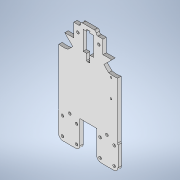
# Autodesk Inventor part: Основа робота
Saved by Autodesk Inventor 2020 (Build 240168000, 168)
## iProperties
Created: 2021-02-28
Part Number: Основа робота
Material: Типовые
Document SubType Name: Обычные детали
Designer: Антон
Density: 1 g/cm^3
Appearance: По умолчанию
Mass: 52.0111 g
Surface Area: 352.197 cm^2
Volume: 52.0111 cm^3
Sheet Metal Rule: По умолчанию
Author: Антон
Autodesk Inventor part; units mm, degrees
note: some values were not read from the file. Chosen so that the rebuilt part matches the saved one: direction of "Рельеф1".
ref_plane "YZ Plane" through (0, 0, 0) normal (1, 0, 0) x (0, 1, 0)
ref_plane "XZ Plane" through (0, 0, 0) normal (0, 1, 0) x (-1, 0, 0)
ref_plane "XY Plane" through (0, 0, 0) normal (0, 0, 1) x (1, 0, 0)
sketch "Эскиз1" plane through (0, 0, 0) normal (0, 0, 1) x (1, 0, 0)
  line L0 (0, 0) -> (35, 0)
  line L1 (35, 0) -> (35, 128.55)
  line L2 (35, 128.55) -> (0, 128.55)
  line L3 (0, 128.55) -> (0, 0)
  line L4 (0, 0) -> (-0.3, 0)
  line L5 (-0.3, 0) -> (-0.3, 30.3)
  line L6 (-0.3, 30.3) -> (0, 30.3)
  line L7 (0, 30.3) -> (0, 0)
  line L8 (-0.3, 0) -> (4.25, 0)
  line L9 (4.25, 0) -> (4.25, 4.55)
  line L10 (4.25, 4.55) -> (4.25, 25.75) construction
  circle A0 centre (4.25, 25.75) radius 1.6
  circle A1 centre (4.25, 4.55) radius 1.6
  line L11 (35, 0) -> (25, 0)
  line L12 (25, 0) -> (25, 33)
  line L13 (25, 33) -> (35, 33)
  line L14 (35, 33) -> (35, 0)
  line L15 (25, 4.55) -> (21, 4.55)
  line L16 (25, 25.75) -> (21, 25.75)
  circle A2 centre (21, 25.75) radius 1.6
  circle A3 centre (21, 4.55) radius 1.6
  line L17 (35, 128.55) -> (35, 128.55)
  line L18 (35, 128.55) -> (18, 128.55)
  line L19 (21, 25.75) -> (21, 4.55) construction
  circle A4 centre (22.55, 120.55) radius 1.6
  line L20 (17.6, 128.55) -> (17.6, 112.55)
  line L21 (17.6, 112.55) -> (0, 112.55)
  line L22 (0, 112.55) -> (0, 129.6)
  line L23 (35, 128.55) -> (25.75, 128.55)
  line L24 (25.75, 128.55) -> (25.75, 133)
  line L25 (25.75, 133) -> (35, 133)
  line L26 (35, 133) -> (35, 128.55)
  line L27 (17.6, 120.55) -> (5.05, 120.55) construction
  line L28 (5.05, 120.55) -> (-3.6474, 111.8526) construction
  line L29 (-3.6474, 111.8526) -> (10.8483, 97.3569)
  circle A5 centre (5.05, 120.55) radius 23.9069
  line L30 (0, 112.55) -> (13, 112.55)
  line L31 (13, 112.55) -> (13, 98.0037)
  line L32 (13, 98.0037) -> (0, 98.0037)
  line L33 (0, 98.0037) -> (0, 112.55)
  line L34 (-3.6474, 111.8526) -> (2.0094, 117.5094)
  line L35 (2.0094, 117.5094) -> (16.5051, 103.0138)
  line L36 (16.5051, 103.0138) -> (10.8483, 97.3569)
  line L37 (10.8483, 97.3569) -> (-3.6474, 111.8526)
  point P0 (0, 30.3)
  point P1 (25, 0)
  point P2 (0, 182.1)
  point P3 (21, 15.15)
  point P4 (4.25, 15.15)
  point P5 (11.6, 112.55)
  point P6 (0, 97.1826)
  point P7 (25.75, 132.5104)
  point P8 (27.5786, 128.55)
  point P9 (25.9614, 133)
  point P10 (27.5786, 128.55)
  point P11 (17.336, 116.55)
  point P12 (17.6, 116.9708)
  point P13 (17.6, 132.1292)
  point P14 (14.4448, 116.55)
  point P15 (0, 108.2052)
  point P16 (10.2015, 98.0037)
  point P17 (6.9689, 112.55)
  point P18 (13, 106.5189)
  point P19 (13, 99.5086)
  dimension "d0" = 35
  dimension "d1" = 128.55
  dimension "d191" = 0.3
  dimension "d192" = 30.3
  dimension "d207" = 4.55
  dimension "d208" = 4.55
  dimension "d209" = 21.2
  dimension "d210" = 10
  dimension "d211" = 33
  dimension "d215" = 4
  dimension "d290" = 3.2
  dimension "d387" = 21.2
  dimension "d418" = 4.55
  dimension "d421" = 3.2
  dimension "d427" = 17.6
  dimension "d428" = 16
  dimension "d433" = 4.95
  dimension "d448" = 9.25
  dimension "d450" = 4.45
  dimension "d493" = 12.55
  dimension "d494" = 12.3
  dimension "d495" = 20.5
  dimension "d496" = 13
  dimension "d499" = 135
  dimension "d500" = 8
  constraints: 76 end point, 14 parallel, 10 perpendicular, 8 horizontal, 7 point on line, 6 centre point, 5 coincident, 3 equal radius, 3 midpoint, 2 collinear, 2 horizontal alignment, 2 point on circle, 1 vertical
  measures "d0" distance of L2.end L1.end
  measures "d1" distance of L1.end L0.end
  measures "d191" distance of L5.end L6.end
  measures "d192" distance of L4.end L5.end
  measures "d207" distance of L4.end L8.end
  measures "d208" distance of L8.end L9.end
  measures "d209" distance of L9.end L10.end
  measures "d210" distance of L12.end L13.end
  measures "d211" distance of L11.end L12.end
  measures "d215" distance of L16.start L16.end
  measures "d290" diameter of A2
  measures "d387" distance of L19.end L19.start
  measures "d418" distance from line of L0 L15.end
  measures "d421" diameter of A4
  measures "d427" distance of L20.end L21.end
  measures "d428" distance of L20.start L20.end
  measures "d433" distance of A4.centre L27.start
  measures "d448" distance of L24.end L25.end
  measures "d450" distance of L23.end L24.end
  measures "d493" distance of L27.start L27.end
  measures "d494" distance of L27.end L28.end
  measures "d495" distance of L28.end L29.end
  measures "d496" distance of L31.end L32.end
  measures "d499" angle of L27 L28
  measures "d500" distance between parallel lines of L37 L35
extrude "Выдавливание1" add sketch "Эскиз1" along normal blind 4 contours L3 A5 L2 L1 L13 L12 L0 | L4 L5 L6 L3 | A5 L2 L24 | L24 L25 L26 L2 A5 | L36 L32 A5 | L2 A5 L31 L36 L35 L21 L20 | L32 L36 L31 | L21 L31 L35
mirror "Зеркальное отражение1" about plane through (35, 33, 0) normal (1, 0, 0)
sketch "Эскиз32" plane through (0, 0, 4) normal (0, 0, 1) x (1, 0, 0)
  line L0 (25, 33) -> (45, 33) projected
  line L1 (25, 0) -> (25, 33) construction
  line L2 (45, 0) -> (45, 33) construction
  line L3 (25, 0) -> (45, 0) construction
  line L4 (35, 0) -> (35, 32.3) construction
  line L5 (12.975, 32.3) -> (57.025, 32.3) construction
  dimension "d501" = 32.3
  dimension "d502" = 44.05
  constraints: 6 end point, 2 midpoint, 1 horizontal, 1 perpendicular, 1 vertical
  measures "d501" distance of L4.start L4.end
  measures "d502" distance of L5.start L5.end
hole "Отверстие14" at (12.975, 32.3, 4) at (57.025, 32.3, 4) direction (0, 0, -1) diameter 3.2 end through all
sketch "Эскиз35" plane through (0, 0, 4) normal (0, 0, 1) x (1, 0, 0)
  line L0 (25.75, 133) -> (44.25, 133) construction
  line L1 (35, 133) -> (35, 83) construction
  line L2 (35, 83) -> (62, 83) construction
  line L3 (62, 72) -> (62, 94) construction
  point P0 (0, 0)
  dimension "d503" = 50
  dimension "d504" = 27
  dimension "d505" = 22
  constraints: 6 end point, 2 midpoint, 2 vertical, 1 horizontal
  measures "d503" distance of L1.start L1.end
  measures "d504" distance of L2.end L1.end
  measures "d505" distance of L3.start L3.end
hole "Отверстие16" at (62, 72, 4) at (62, 94, 4) direction (0, 0, -1) diameter 2.2 end through all
sketch "Эскиз33" plane through (0, 0, 4) normal (0, 0, 1) x (1, 0, 0)
  line L0 (25.75, 133) -> (35, 133) construction
  line L1 (35, 133) -> (35, 129) construction
  line L2 (41.25, 127) -> (28.75, 127)
  line L3 (28.75, 127) -> (28.75, 104.2)
  line L4 (28.75, 104.2) -> (41.25, 104.2)
  line L5 (41.25, 104.2) -> (41.25, 127)
  line L6 (33, 129) -> (37, 129)
  line L7 (37, 129) -> (37, 127)
  line L8 (37, 127) -> (33, 127)
  line L9 (33, 127) -> (33, 129)
  line L10 (33, 104.2) -> (37, 104.2)
  line L11 (37, 104.2) -> (37, 96)
  line L12 (37, 96) -> (33, 96)
  line L13 (33, 96) -> (33, 104.2)
  point P0 (0, 0)
  point P1 (44.25, 133)
  point P2 (35, 127)
  point P3 (35, 104.2)
  point P4 (37, 127)
  point P5 (33, 127)
  point P6 (26.4635, 133)
  dimension "d465" = 12.5
  dimension "d466" = 22.8
  dimension "d467" = 2
  dimension "d468" = 4
  dimension "d469" = 4
  dimension "d470" = 4
  dimension "d471" = 8.2
  constraints: 27 end point, 6 parallel, 5 midpoint, 3 horizontal, 3 perpendicular, 1 vertical
  measures "d465" distance between parallel lines of L5 L3
  measures "d466" distance of L4.end L2.start
  measures "d467" distance of L6.end L7.end
  measures "d468" distance of L6.start L6.end
  measures "d469" distance of L0.end L1.end
  measures "d470" distance of L11.end L12.end
  measures "d471" distance of L10.end L11.end
extrude "Выдавливание14" cut sketch "Эскиз33" against normal through all
fillet "Сопряжение14" radius 1 2 edges at (37, 96, 2) (33, 96, 2)
fillet "Сопряжение13" radius 2.225 4 edges at (25.75, 128.55, 2) (25.75, 133, 2) (44.25, 128.55, 2) (44.25, 133, 2)
fillet "Сопряжение2" radius 5.05 6 edges at (-0.3, 30.3, 2) (-0.3, 0, 2) (25, 0, 2) (45, 0, 2) (70.3, 0, 2) (70.3, 30.3, 2)
sketch "Эскиз19" plane through (0, 0, 0) normal (0, 0, -1) x (-1, 0, 0)
  line L0 (-25.75, 128.55) -> (-17.6, 128.55) projected
  line L1 (-25.35, 122.1666) -> (-22.55, 123.7832)
  line L2 (-22.55, 123.7832) -> (-19.75, 122.1666)
  line L3 (-19.75, 122.1666) -> (-19.75, 118.9334)
  line L4 (-19.75, 118.9334) -> (-22.55, 117.3168)
  line L5 (-22.55, 117.3168) -> (-25.35, 118.9334)
  line L6 (-25.35, 118.9334) -> (-25.35, 122.1666)
  line L7 (0, 97.1826) -> (0, 30.3) projected
  circle A0 centre (-22.55, 120.55) radius 1.6 projected
  point P0 (0, 128.55)
  point P1 (-70, 128.55)
  point P2 (-14, 129.6)
  point P3 (-64, 129.6)
  point P4 (0, 119.25)
  point P5 (0, 116.55)
  point P6 (0, 129.6)
  point P7 (-78, 129.6)
  point P8 (-17.6, 128.55)
  point P9 (-52.4, 128.55)
  point P10 (0, 107.125)
  point P11 (-35, 132.55)
  point P12 (-27.0423, 128.55)
  point P13 (0, 0)
  point P14 (0, 102.0037)
  dimension "d423" = 5.6
  constraints: 12 end point, 1 coincident, 1 vertical, 15 other
  measures "d423" distance between parallel lines of L3 L6
extrude "Выдавливание7" cut sketch "Эскиз19" against normal blind 2.6 contours L1 L2 L3 L4 L5 L6 | A0
sketch "Эскиз25" plane through (0, 0, 0) normal (0, 0, -1) x (-1, 0, 0)
  circle A0 centre (-21, 25.75) radius 1.6 projected
  circle A1 centre (-21, 4.55) radius 1.6 projected
  circle A2 centre (-4.25, 25.75) radius 1.6 projected
  circle A3 centre (-4.25, 4.55) radius 1.6 projected
  circle A4 centre (-49, 25.75) radius 1.6 projected
  circle A5 centre (-49, 4.55) radius 1.6 projected
  circle A6 centre (-65.75, 4.55) radius 1.6 projected
  circle A7 centre (-65.75, 25.75) radius 1.6 projected
  circle A8 centre (-47.45, 120.55) radius 1.6 projected
  circle A9 centre (-47.45, 120.55) radius 1.6 projected
  circle A10 centre (-57.025, 32.3) radius 1.6 projected
  circle A11 centre (-12.975, 32.3) radius 1.6 projected
  circle A12 centre (-57.025, 32.3) radius 1.6 projected
  circle A13 centre (-12.975, 32.3) radius 1.6 projected
  point P0 (0, 0)
  constraints: 12 coincident
pattern_sketch "Массив по эскизу1" of "Выдавливание7" from (22.55, 120.55, 0) copies at (21, 25.75, 0) at (21, 4.55, 0) at (4.25, 25.75, 0) at (4.25, 4.55, 0) at (49, 25.75, 0) at (49, 4.55, 0) at (65.75, 4.55, 0) at (65.75, 25.75, 0) at (47.45, 120.55, 0) at (57.025, 32.3, 0) at (12.975, 32.3, 0)
sketch "Эскиз31" plane through (0, 0, 0) normal (0, 0, -1) x (-1, 0, 0)
  line L0 (-70, 96.6431) -> (0, 96.6431) construction
  line L1 (0, 96.6431) -> (0, 33) construction
  line L2 (0, 33) -> (-70, 33) construction
  line L3 (-70, 33) -> (-70, 96.6431) construction
  line L4 (0, 97.1826) -> (0, 30.3) projected
  line L5 (-70, 97.1826) -> (-70, 30.3) projected
  line L6 (-25, 33) -> (-45, 33) projected
  arc A0 (-10.8483, 97.3569) -> (0, 97.1826) centre (-5.05, 120.55) ccw projected
  line L7 (-43.3655, 68.2237) -> (-41.8166, 72.9961)
  line L8 (-41.8166, 72.9961) -> (-40.6499, 72.9961)
  line L9 (-40.6499, 72.9961) -> (-42.8475, 66.8961)
  line L10 (-42.8475, 66.8961) -> (-43.8734, 66.8961)
  line L11 (-43.8734, 66.8961) -> (-46.061, 72.9961)
  line L12 (-46.061, 72.9961) -> (-44.8993, 72.9961)
  line L13 (-44.8993, 72.9961) -> (-43.3655, 68.2237)
  line L14 (-38.9803, 66.8961) -> (-39.9962, 66.8961)
  line L15 (-39.9962, 66.8961) -> (-39.9962, 71.4271)
  line L16 (-39.9962, 71.4271) -> (-38.9803, 71.4271)
  line L17 (-38.9803, 71.4271) -> (-38.9803, 66.8961)
  spline S0 degree 2 poles (-40.0615, 72.6038) (-40.0615, 72.8352) (-39.7648, 73.1469) (-39.2117, 73.1469) (-38.9099, 72.8352) (-38.9099, 72.6038) knots 0 0 0 1 2 3 4 4 4
  spline S1 degree 2 poles (-38.9099, 72.6038) (-38.9099, 72.3725) (-39.2117, 72.0657) (-39.7648, 72.0657) (-40.0615, 72.3725) (-40.0615, 72.6038) knots 0 0 0 1 2 3 4 4 4
  spline S2 degree 2 poles (-38.0601, 69.2043) (-38.0601, 69.8681) (-37.532, 70.9393) (-36.5765, 71.5126) (-35.958, 71.5126) knots 0 0 0 1 2 3 3 3
  spline S3 degree 2 poles (-35.958, 71.5126) (-35.0427, 71.5126) (-33.8962, 70.3308) (-33.8509, 69.3552) knots 0 0 0 1 2 2 2
  line L18 (-33.8509, 69.3552) -> (-33.8459, 69.1138)
  spline S4 degree 2 poles (-33.8459, 69.1138) (-33.8459, 68.445) (-34.3639, 67.3889) (-35.3244, 66.8106) (-35.9479, 66.8106) knots 0 0 0 1 2 3 3 3
  spline S5 degree 2 poles (-35.9479, 66.8106) (-36.9085, 66.8106) (-38.0601, 68.0879) (-38.0601, 69.154) knots 0 0 0 1 2 2 2
  line L19 (-38.0601, 69.154) -> (-38.0601, 69.2043)
  spline S6 degree 2 poles (-37.0442, 69.1188) (-37.0442, 68.4198) (-36.4659, 67.6253) (-35.435, 67.6253) (-34.8617, 68.4299) (-34.8617, 69.2043) knots 0 0 0 1 2 3 4 4 4
  spline S7 degree 2 poles (-34.8617, 69.2043) (-34.8617, 69.8933) (-35.4501, 70.6979) (-35.958, 70.6979) knots 0 0 0 1 2 2 2
  spline S8 degree 2 poles (-35.958, 70.6979) (-36.4559, 70.6979) (-37.0442, 69.9033) (-37.0442, 69.1188) knots 0 0 0 1 2 2 2
  line L20 (-31.9047, 66.8961) -> (-32.9206, 66.8961)
  line L21 (-32.9206, 66.8961) -> (-32.9206, 73.333)
  line L22 (-32.9206, 73.333) -> (-31.9047, 73.333)
  line L23 (-31.9047, 73.333) -> (-31.9047, 66.8961)
  spline S9 degree 2 poles (-28.8019, 66.8106) (-29.7675, 66.8106) (-30.9694, 68.0326) (-30.9694, 69.0434) knots 0 0 0 1 2 2 2
  line L24 (-30.9694, 69.0434) -> (-30.9694, 69.1691)
  spline S10 degree 2 poles (-30.9694, 69.1691) (-30.9694, 69.848) (-30.4464, 70.9192) (-29.5009, 71.5126) (-28.9176, 71.5126) knots 0 0 0 1 2 3 3 3
  spline S11 degree 2 poles (-28.9176, 71.5126) (-27.9923, 71.5126) (-26.9815, 70.3308) (-26.9815, 69.2546) knots 0 0 0 1 2 2 2
  line L25 (-26.9815, 69.2546) -> (-26.9815, 68.8422)
  line L26 (-26.9815, 68.8422) -> (-29.9435, 68.8422)
  spline S12 degree 2 poles (-29.9435, 68.8422) (-29.8982, 68.279) (-29.2394, 67.6253) (-28.7416, 67.6253) knots 0 0 0 1 2 2 2
  spline S13 degree 2 poles (-28.7416, 67.6253) (-28.0426, 67.6253) (-27.6, 68.1885) knots 0 0 0 1 1 1
  line L27 (-27.6, 68.1885) -> (-27.0519, 67.6655)
  spline S14 degree 2 poles (-27.0519, 67.6655) (-27.3235, 67.2582) (-28.2337, 66.8106) (-28.8019, 66.8106) knots 0 0 0 1 2 2 2
  spline S15 degree 2 poles (-28.9226, 70.6979) (-29.34, 70.6979) (-29.858, 70.1095) (-29.9284, 69.5865) knots 0 0 0 1 2 2 2
  line L28 (-29.9284, 69.5865) -> (-27.9873, 69.5865)
  line L29 (-27.9873, 69.5865) -> (-27.9873, 69.662)
  spline S16 degree 2 poles (-27.9873, 69.662) (-28.0225, 70.1749) (-28.5002, 70.6979) (-28.9226, 70.6979) knots 0 0 0 1 2 2 2
  line L30 (-24.9197, 72.5284) -> (-24.9197, 71.4271)
  line L31 (-24.9197, 71.4271) -> (-24.1201, 71.4271)
  line L32 (-24.1201, 71.4271) -> (-24.1201, 70.6728)
  line L33 (-24.1201, 70.6728) -> (-24.9197, 70.6728)
  line L34 (-24.9197, 70.6728) -> (-24.9197, 68.1432)
  spline S17 degree 2 poles (-24.9197, 68.1432) (-24.9197, 67.8817) (-24.7135, 67.6504) (-24.452, 67.6504) knots 0 0 0 1 2 2 2
  spline S18 degree 2 poles (-24.452, 67.6504) (-24.276, 67.6504) (-24.0949, 67.6906) knots 0 0 0 1 1 1
  line L35 (-24.0949, 67.6906) -> (-24.0949, 66.9061)
  spline S19 degree 2 poles (-24.0949, 66.9061) (-24.4419, 66.8106) (-24.7638, 66.8106) knots 0 0 0 1 1 1
  spline S20 degree 2 poles (-24.7638, 66.8106) (-25.9355, 66.8106) (-25.9355, 68.103) knots 0 0 0 1 1 1
  line L36 (-25.9355, 68.103) -> (-25.9355, 70.6728)
  line L37 (-25.9355, 70.6728) -> (-26.6798, 70.6728)
  line L38 (-26.6798, 70.6728) -> (-26.6798, 71.4271)
  line L39 (-26.6798, 71.4271) -> (-25.9355, 71.4271)
  line L40 (-25.9355, 71.4271) -> (-25.9355, 72.5284)
  line L41 (-25.9355, 72.5284) -> (-24.9197, 72.5284)
  line L42 (-45.2488, 62.4553) -> (-43.4937, 57.7785)
  line L43 (-43.4937, 57.7785) -> (-41.7387, 62.4553)
  line L44 (-41.7387, 62.4553) -> (-40.3658, 62.4553)
  line L45 (-40.3658, 62.4553) -> (-40.3658, 56.3553)
  line L46 (-40.3658, 56.3553) -> (-41.4218, 56.3553)
  line L47 (-41.4218, 56.3553) -> (-41.4218, 58.3669)
  line L48 (-41.4218, 58.3669) -> (-41.3162, 61.0573)
  line L49 (-41.3162, 61.0573) -> (-43.1166, 56.3553)
  line L50 (-43.1166, 56.3553) -> (-43.8759, 56.3553)
  line L51 (-43.8759, 56.3553) -> (-45.6763, 61.0523)
  line L52 (-45.6763, 61.0523) -> (-45.5707, 58.3669)
  line L53 (-45.5707, 58.3669) -> (-45.5707, 56.3553)
  line L54 (-45.5707, 56.3553) -> (-46.6267, 56.3553)
  line L55 (-46.6267, 56.3553) -> (-46.6267, 62.4553)
  line L56 (-46.6267, 62.4553) -> (-45.2488, 62.4553)
  line L57 (-37.7357, 58.2965) -> (-38.1883, 57.8338)
  line L58 (-38.1883, 57.8338) -> (-38.1883, 56.3553)
  line L59 (-38.1883, 56.3553) -> (-39.2092, 56.3553)
  line L60 (-39.2092, 56.3553) -> (-39.2092, 62.7923)
  line L61 (-39.2092, 62.7923) -> (-38.1883, 62.7923)
  line L62 (-38.1883, 62.7923) -> (-38.1883, 59.076)
  line L63 (-38.1883, 59.076) -> (-37.8715, 59.4732)
  line L64 (-37.8715, 59.4732) -> (-36.6193, 60.8863)
  line L65 (-36.6193, 60.8863) -> (-35.3973, 60.8863)
  line L66 (-35.3973, 60.8863) -> (-37.0819, 58.9955)
  line L67 (-37.0819, 58.9955) -> (-35.2162, 56.3553)
  line L68 (-35.2162, 56.3553) -> (-36.393, 56.3553)
  line L69 (-36.393, 56.3553) -> (-37.7357, 58.2965)
  spline S21 degree 2 poles (-34.0998, 57.4265) (-33.8182, 57.4265) (-33.5064, 57.1046) (-33.5064, 56.8633) knots 0 0 0 1 2 2 2
  spline S22 degree 2 poles (-33.5064, 56.8633) (-33.5064, 56.6219) (-33.8182, 56.3101) (-34.0998, 56.3101) knots 0 0 0 1 2 2 2
  spline S23 degree 2 poles (-34.0998, 56.3101) (-34.3714, 56.3101) (-34.6932, 56.6219) (-34.6932, 57.1046) (-34.3815, 57.4265) (-34.0998, 57.4265) knots 0 0 0 1 2 3 4 4 4
  line L70 (-28.9855, 56.3553) -> (-30.0416, 56.3553)
  line L71 (-30.0416, 56.3553) -> (-30.0416, 62.4553)
  line L72 (-30.0416, 62.4553) -> (-28.9855, 62.4553)
  line L73 (-28.9855, 62.4553) -> (-28.9855, 56.3553)
  line L74 (-25.5357, 57.683) -> (-23.9868, 62.4553)
  line L75 (-23.9868, 62.4553) -> (-22.8201, 62.4553)
  line L76 (-22.8201, 62.4553) -> (-25.0177, 56.3553)
  line L77 (-25.0177, 56.3553) -> (-26.0436, 56.3553)
  line L78 (-26.0436, 56.3553) -> (-28.2312, 62.4553)
  line L79 (-28.2312, 62.4553) -> (-27.0695, 62.4553)
  line L80 (-27.0695, 62.4553) -> (-25.5357, 57.683)
  point P0 (-70, 0)
  constraints: 3 collinear, 1 tangent, 2 other
emboss "Рельеф1" sketch "Эскиз31" operation cut depth 0.5 direction (0, 0, 1)
equation "\"Радиус_гибки\" = Толщина"
equation "\"Ширина_просечки\" = Толщина"
equation "\"Глубина_просечки\" = 0.5 * Толщина"
equation "\"Размер_просечки\" = 4 * Толщина"
equation "\"Мин_остаток\" = 2 * Толщина"
equation "\"Радиус_перехода\" = Радиус_гибки"
equation "\"Радиус_Якоби\" = Толщина"
equation "\"Размер_зазора\" = Толщина"
equation "\"Гайка_М3_з\" = 5.6"
equation "\"d130\" = 5.6"
equation "\"Толщина\" = 0.5"
